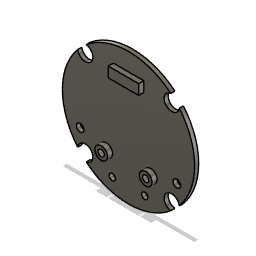
Base Plate (Autodesk Fusion 360 design; units mm, degrees)
Autodesk Fusion 360 part; units mm, degrees
sketch "Sketch1" plane through (0, 0, 0) normal (0, 0, 1) x (1, 0, 0)
  line L0 (17, -17) -> (-17, -17) construction
  line L1 (-17, -17) -> (-17, 17) construction
  line L2 (-17, 17) -> (17, 17) construction
  line L3 (17, 17) -> (17, -17) construction
  line L4 (17, -17) -> (-17, 17) construction
  line L5 (-17, -17) -> (17, 17) construction
  circle A0 centre (17, -17) radius 3
  circle A1 centre (17, 17) radius 3
  circle A2 centre (-17, 17) radius 3
  circle A3 centre (-17, -17) radius 3
  line L6 (-19, -9.5) -> (19, -9.5) construction
  circle A4 centre (19, -9.5) radius 1.5
  circle A5 centre (-19, -9.5) radius 1.5
  circle A6 centre (0, 0) radius 26
  dimension "d1" = 34
  dimension "d2" = 34
  dimension "d3" = 6
  dimension "d4" = 6
  dimension "d5" = 6
  dimension "d6" = 6
  dimension "d7" = 38
  dimension "d8" = 7.5
  dimension "d9" = 3
  dimension "d10" = 3
  dimension "d11" = 52
  constraint horizontal L0
  constraint perpendicular L0 L1
  constraint parallel L1 L3
  constraint coincident L0.start L3.end
  constraint coincident L2.end L3.start
  constraint coincident L1.end L2.start
  constraint coincident L0.end L1.start
  constraint perpendicular L1 L6
  constraint coincident L6.end A4.centre
  constraint coincident L6.start A5.centre
  measures "d1" distance of L1.end L2.end
  measures "d2" distance of L0.end L1.end
  measures "d3" diameter of A0
  measures "d4" diameter of A1
  measures "d5" diameter of A2
  measures "d6" diameter of A3
  measures "d7" distance of L6.start L6.end
  measures "d8" distance of L0 L6
  measures "d9" diameter of A4
  measures "d10" diameter of A5
  measures "d11" diameter of A6
extrude "Extrude1" add sketch "Sketch1" along normal blind 1.6 contours A0 A1 A2 A3 A6
sketch "Sketch2" plane through (0, 0, 1.6) normal (0, 0, 1) x (1, 0, 0)
  circle A0 centre (-19, -9.5) radius 1.5
  circle A1 centre (19, -9.5) radius 1.5
  line L0 (6, 19) -> (6, 15)
  line L1 (-6, 19) -> (6, 19)
  circle A2 centre (8.75, -12) radius 1.25
  line L2 (6, 15) -> (-6, 19) construction
  circle A3 centre (8.75, -12) radius 2.5
  circle A4 centre (-8.75, -12) radius 2.5
  line L3 (-6, 15) -> (6, 19) construction
  line L4 (6, 15) -> (-6, 15)
  line L5 (-6, 15) -> (-6, 19)
  line L6 (-8.75, -12) -> (8.75, -12) construction
  circle A5 centre (-8.75, -12) radius 1.25
  line L7 (0, 30) -> (0, -30) construction
  point P0 (0, 17)
  point P1 (0, -12)
  dimension "d23" = 12
  dimension "d24" = 4
  dimension "d25" = 17.5
  dimension "d26" = 2.5
  dimension "d27" = 5
  dimension "d28" = 5
  dimension "d29" = 2.5
  constraint horizontal L4
  constraint perpendicular L4 L5
  constraint parallel L1 L4
  constraint parallel L0 L5
  constraint coincident P0 L2
  constraint coincident P0 L3
  constraint coincident P1 L6
  constraint midpoint P1 L6
  constraint coincident A2.centre A3.centre
  constraint concentric A2 A3
  constraint coincident A4.centre L6.start
  constraint concentric A4 A5
  constraint perpendicular L4 L7
  constraint coincident P1 L7
  measures "d23" distance of L0.start L1.start
  measures "d24" distance of L3.start L1.start
  measures "d25" distance of A4.centre A2.centre
  measures "d26" diameter of A2
  measures "d27" diameter of A3
  measures "d28" diameter of A4
  measures "d29" diameter of A5
extrude "Extrude2" add sketch "Sketch2" along normal blind 2 contours L0 L1 L4 L5 | A3 | A4
extrude "Extrude3" cut sketch "Sketch2" against normal blind 2 contours A2 | A5
sketch "Sketch3" plane through (0, 0, 1.6) normal (0, 0, 1) x (1, 0, 0)
  line L0 (-6, 15) -> (-6, 19)
  line L1 (-6, 19) -> (6, 19)
  line L2 (6, 19) -> (6, 15)
  line L3 (6, 15) -> (-6, 15)
  circle A0 centre (8.75, -12) radius 2.5
  circle A1 centre (-19, -9.5) radius 1.5
  circle A2 centre (19, -9.5) radius 1.5
  arc A3 (-16.6394, -19.9782) -> (16.6394, -19.9782) centre (0, 0) ccw
  arc A4 (19.9782, -16.6394) -> (16.6394, -19.9782) centre (17, -17) ccw
  arc A5 (19.9782, -16.6394) -> (19.9782, 16.6394) centre (0, 0) ccw
  arc A6 (16.6394, 19.9782) -> (19.9782, 16.6394) centre (17, 17) ccw
  arc A7 (16.6394, 19.9782) -> (-16.6394, 19.9782) centre (0, 0) ccw
  arc A8 (-19.9782, 16.6394) -> (-16.6394, 19.9782) centre (-17, 17) ccw
  arc A9 (-19.9782, 16.6394) -> (-19.9782, -16.6394) centre (0, 0) ccw
  arc A10 (-16.6394, -19.9782) -> (-19.9782, -16.6394) centre (-17, -17) ccw
  circle A11 centre (-8.75, -12) radius 2.5
  line L4 (-6.375, -20) -> (6.375, -20)
  circle A12 centre (6.375, -20) radius 1.25
  circle A13 centre (-6.375, -20) radius 1.25
  point P0 (0, -20)
  point P1 (8.75, -12)
  dimension "d36" = 12.75
  dimension "d37" = 8
  dimension "d38" = 2.5
  dimension "d39" = 2.5
  constraint horizontal L4
  constraint coincident L4 P0
  constraint midpoint L4 P0
  constraint coincident L4.end A12.centre
  constraint coincident L4.start A13.centre
  measures "d36" distance of L4.start L4.end
  measures "d37" distance of L4 P1
  measures "d38" diameter of A12
  measures "d39" diameter of A13
extrude "Extrude5" cut sketch "Sketch3" against normal through all contours A12 | A13
named bodies: "Base Plate"
